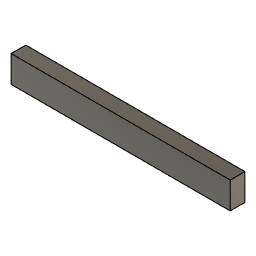
多分教室上の配管通ってるやつ[550と1000の値は流用可能] (Autodesk Fusion 360 design; units mm, degrees)
Autodesk Fusion 360 part; units mm, degrees
sketch "スケッチ1" plane through (0, 0, 0) normal (0, 0, 1) x (1, 0, 0)
  line L0 (0, 0) -> (8210, 0)
  line L1 (8210, 0) -> (8210, 550)
  line L2 (8210, 550) -> (0, 550)
  line L3 (0, 550) -> (0, 0)
  dimension "d1" = 8210
  dimension "d2" = 550
  constraint horizontal L0
  constraint vertical L1
  constraint horizontal L2
  constraint vertical L3
  constraint coincident L0.start L3.end
  measures "d1" distance of L0.start L0.end
  measures "d2" distance of L0.start L2.end
extrude "押し出し1" add sketch "スケッチ1" along normal blind 1000
